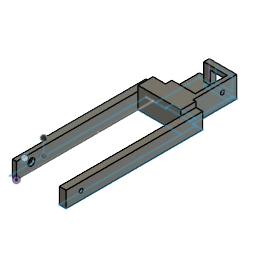
Davinki Bicep (Autodesk Fusion 360 design; units mm, degrees)
part number: 2026-09-06-07-50-14-752
Autodesk Fusion 360 part; units mm, degrees
note: some values were not read from the file. Chosen so that the rebuilt part matches the saved one: which face or edge a step refers to. Set by a fixed rule: which sketch regions a step uses.
sketch "Sketch1" plane through (0, 0, 0) normal (0, 1, 0) x (1, 0, 0)
  line L0 (0, 0) -> (0, 60)
  line L1 (31.4, 0) -> (31.4, 60)
  line L2 (0, 60) -> (0, 100)
  line L3 (31.4, 60) -> (31.4, 100)
  line L4 (31.4, 0) -> (36.4, 0)
  line L5 (36.4, 0) -> (36.4, 100)
  line L6 (36.4, 100) -> (31.4, 100)
  line L7 (0, 100) -> (-5, 100)
  line L8 (-5, 100) -> (-5, 0)
  line L9 (-5, 0) -> (0, 0)
  line L10 (2.05, 124) -> (2.05, 100.6)
  line L11 (26.35, 124) -> (26.35, 100.6)
  line L12 (26.35, 100.6) -> (26.35, 104.6)
  line L13 (2.05, 100.6) -> (2.05, 100)
  line L14 (2.05, 100) -> (0, 100)
  line L15 (29.35, 100.6) -> (29.35, 100)
  line L16 (29.35, 100) -> (31.4, 100)
  line L17 (0, 89) -> (31.4, 89)
  line L18 (29.35, 100.6) -> (29.35, 132)
  line L19 (29.35, 132) -> (2.05, 132)
  line L20 (2.05, 132) -> (2.05, 124)
  line L21 (26.35, 124) -> (26.35, 132)
  line L22 (26.35, 132) -> (26.35, 128)
  line L23 (6.35, 100) -> (2.05, 100)
  line L24 (26.35, 100.6) -> (9.15, 100.6)
  line L25 (26.35, 128) -> (9.15, 128)
  line L26 (26.35, 104.6) -> (9.15, 104.6)
  line L27 (9.15, 100.6) -> (9.15, 104.6)
  line L28 (9.15, 128) -> (9.15, 132)
  line L29 (6.35, 100) -> (9.15, 100)
  line L30 (9.15, 100) -> (9.15, 100.6)
  dimension "d1" = 60
  dimension "d2" = 31.4
  dimension "d4" = 40
  dimension "d6" = 5
  dimension "d25" = 31.4
  dimension "d26" = 27.3
  dimension "d27" = 4
  dimension "d82" = 17.2
  dimension "d83" = 17.2
  dimension "d84" = 17.2
  constraint coincident L0.start L9.end
  constraint vertical L0
  constraint parallel L0 L2
  constraint parallel L1 L3
  constraint perpendicular L3 L4
  constraint perpendicular L4 L5
  constraint perpendicular L5 L6
  constraint perpendicular L2 L7
  constraint perpendicular L6 L8
  constraint perpendicular L0 L9
  constraint coincident L2 L17.start
  constraint coincident L3 L17.end
  constraint perpendicular L3 L17
  constraint perpendicular L18 L19
  constraint perpendicular L19 L20
  constraint coincident L19 L21.end
  constraint perpendicular L19 L21
  constraint perpendicular L19 L22
  constraint perpendicular L13 L23
  constraint perpendicular L11 L24
  constraint perpendicular L22 L25
  constraint perpendicular L11 L26
  constraint perpendicular L26 L27
  constraint coincident L19 L28.end
  constraint perpendicular L19 L28
  constraint perpendicular L27 L29
  constraint perpendicular L24 L30
  measures "d1" distance of L0.start L0.end
  measures "d2" distance of L0.start L1.start
  measures "d4" distance of L0.end L2.end
  measures "d6" distance of L1.start L4.end
  measures "d25" distance of L15.start L18.end
  measures "d26" distance of L18.end L19.end
  measures "d27" distance of L21.end L22.end
  measures "d82" distance of L11.end L24.end
  measures "d83" distance of L22.end L25.end
  measures "d84" distance of L12.end L26.end
extrude "Extrude2" add sketch "Sketch1" along normal blind 11.6 contours L0 L2 L7 L8 L9 | L2 L3 L11 L12 L14 L15 L16 L17 L18 L19 L21 L22 L23 L24 L29 L30 | L1 L3 L4 L5 L6
extrude "Extrude5" add sketch "Sketch1" along normal blind 3 contours L10 L11 L13 L19 L20 L21 L23 L25 L26 L27 L28 L29 L30
extrude "Extrude6" add sketch "Sketch1" along normal blind 15.5 contours L2 L3 L11 L12 L14 L15 L16 L17 L18 L19 L21 L22 L23 L24 L29 L30 | L11 L12 L24 L26 L27 | L19 L21 L22 L25 L28
sketch "Sketch2" plane through (0, 0, -132) normal (0, 0, -1) x (-1, 0, 0)
  line L0 (-29.35, 0) -> (-2.05, 0)
  line L1 (-2.05, 0) -> (-2.05, 3)
  line L2 (-2.05, 3) -> (-9.15, 3)
  line L3 (-9.15, 15.5) -> (-29.35, 15.5)
  line L4 (-29.35, 15.5) -> (-29.35, 0)
  line L5 (-26, 12.5) -> (-14, 12.5)
  line L6 (-14, 12.5) -> (-14, 3)
  line L7 (-14, 3) -> (-26, 3)
  line L8 (-26, 3) -> (-26, 12.5)
  line L9 (-9.15, 3) -> (-9.15, 15.5)
  constraint horizontal L5
  constraint vertical L6
  constraint horizontal L7
  constraint vertical L8
extrude "Extrude7" cut sketch "Sketch2" against normal blind 16 contours L5 L6 L7 L8
sketch "Sketch3" plane through (-5, 0, 0) normal (-1, 0, 0) x (0, 0, 1)
  line L0 (-100, 0) -> (0, 0)
  line L1 (0, 0) -> (0, 11.6)
  line L2 (0, 11.6) -> (-100, 11.6)
  line L3 (-100, 11.6) -> (-100, 0)
  line L4 (-25, 0) -> (-25, 11.6)
  circle A0 centre (-11, 5.8) radius 1.2
  circle A1 centre (-11, 5.8) radius 2.5
  dimension "d35" = 2.4
  dimension "d50" = 5
  constraint coincident L0 L4.start
  constraint coincident L2 L4.end
  constraint perpendicular L2 L4
  constraint concentric A0 A1
  measures "d35" diameter of A0
  measures "d50" diameter of A1
extrude "Extrude8" cut sketch "Sketch3" against normal blind 2 contours L0 L1 L2 L4 | A1
sketch "Sketch4" plane through (36.4, 0, 0) normal (1, 0, 0) x (0, 0, -1)
  line L0 (0, 0) -> (100, 0)
  line L1 (100, 0) -> (100, 11.6)
  line L2 (100, 11.6) -> (0, 11.6)
  line L3 (0, 11.6) -> (0, 0)
  line L4 (25, 11.6) -> (25, 0)
  line L5 (11, 0) -> (11, 5.8)
  constraint coincident L2 L4.start
  constraint coincident L0 L4.end
  constraint perpendicular L0 L4
  constraint coincident L0 L5.start
  constraint perpendicular L0 L5
hole "Hole1" at (36.4, 5.8, -11) direction (-1, 0, 0) diameter 2.7 depth 4.5 tip angle 118
extrude "Extrude9" cut sketch "Sketch3" against normal blind 10 contours A0
extrude "Extrude10" cut sketch "Sketch3" against normal blind 6 contours A1
extrude "Extrude11" add sketch "Sketch3" against normal blind 4 contours A1
extrude "Extrude12" cut sketch "Sketch3" against normal blind 2 contours A1
extrude "Extrude13" cut sketch "Sketch3" against normal blind 16 contours A1
extrude "Extrude14" add sketch "Sketch3" against normal blind 3 contours A1
extrude "Extrude15" cut sketch "Sketch3" against normal blind 2 contours A1
sketch "Sketch5" plane through (0, 0, 0) normal (1, 0, 0) x (0, 0, -1)
sketch "Sketch6" plane through (6.35, 0, 0) normal (-1, 0, 0) x (0, 0, 1)
  line L0 (-104.6, 3) -> (-100.6, 3)
  line L1 (-100.6, 15.5) -> (-104.6, 15.5)
  line L2 (-104.6, 15.5) -> (-104.6, 3)
  line L3 (-102.6, 3) -> (-102.6, 9.25)
  line L4 (-100.6, 3) -> (-100.6, 11.6)
  line L5 (-100.6, 11.6) -> (-100.6, 15.5)
  constraint midpoint L0 L3.start
  constraint perpendicular L0 L3
hole "Hole2" at (6.35, 9.25, -102.6) direction (1, 0, 0) diameter 2.076 depth 7 tip angle 180
thread "Thread1" "ISO Metric profile 2.5 M2.5x0.45 M2.5x0.45 6H" thread offset 0 thread depth 7.4
sketch "Sketch7" plane through (6.35, 0, 0) normal (-1, 0, 0) x (0, 0, 1)
  line L0 (-132, 3) -> (-128, 3)
  line L1 (-128, 3) -> (-128, 15.5)
  line L2 (-128, 15.5) -> (-132, 15.5)
  line L3 (-132, 15.5) -> (-132, 3)
  line L4 (-132, 3) -> (-130, 3)
  line L5 (-130, 3) -> (-130, 9.25)
  dimension "d68" = 2
  dimension "d69" = 6.25
  constraint coincident L0.start L3.end
  constraint perpendicular L3 L4
  constraint perpendicular L4 L5
  measures "d68" distance of L0.start L4.end
  measures "d69" distance of L4.end L5.end
hole "Hole3" at (6.35, 9.25, -130) direction (1, 0, 0) diameter 2.076 depth 6.5 tip angle 180
thread "Thread2" "ISO Metric profile 2.5 M2.5x0.45 M2.5x0.45 6H" thread offset 0 thread depth 7.4
sketch "Sketch8" plane through (29.35, 0, 0) normal (1, 0, 0) x (0, 0, -1)
  line L0 (100, 15.5) -> (100, 0)
  line L1 (100, 0) -> (132, 0)
  line L2 (132, 0) -> (132, 15.5)
  line L3 (132, 15.5) -> (100, 15.5)
  line L4 (100, 15.5) -> (100, 0)
  line L5 (117, 9.25) -> (104.6, 9.25)
  line L6 (104.6, 9.25) -> (121.5, 9.25)
  dimension "d78" = 16.9
  constraint coincident L0.start L3.end
  constraint coincident L1 L0.end
  constraint perpendicular L1 L4
  measures "d78" distance of L5.end L6.end
hole "Hole4" at (29.35, 9.25, -121.5) direction (-1, 0, 0) diameter 2.8 depth 2.5 tip angle 180
